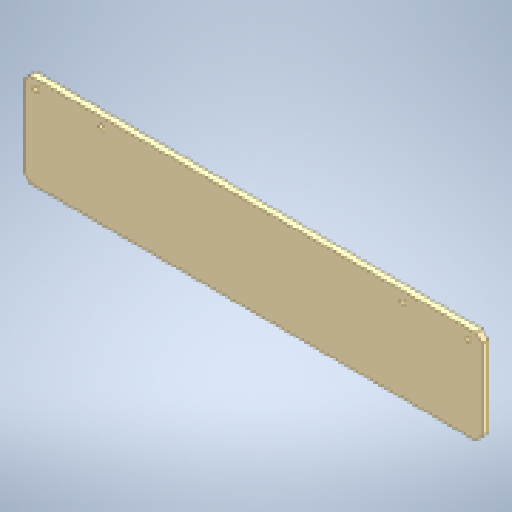
# Autodesk Inventor part: фанера_для_электр
Saved by Autodesk Inventor 2023.1 (Build 271208000, 208)
## iProperties
Created: 2026-01-13
Part Number: фанера_для_электр
Material: Типовые
Document SubType Name: Modeling
Designer: DELL
Density: 1 g/cm^3
Appearance: Бежевый
Author: DELL
Autodesk Inventor part; units mm, degrees
ref_plane "YZ Plane" through (0, 0, 0) normal (1, 0, 0) x (0, 1, 0)
ref_plane "XZ Plane" through (0, 0, 0) normal (0, 1, 0) x (-1, 0, 0)
ref_plane "XY Plane" through (0, 0, 0) normal (0, 0, 1) x (1, 0, 0)
sketch "Эскиз1" plane through (0, 0, 0) normal (0, 0, 1) x (1, 0, 0)
  line L0 (-286.7881, 32) -> (-6.2881, 32)
  line L1 (-6.2881, 32) -> (-6.2881, -25)
  line L2 (-6.2881, -25) -> (-286.7881, -25)
  line L3 (-286.7881, -25) -> (-286.7881, 32)
  line L4 (-286.7881, 32) -> (-6.2881, -25) construction
  line L5 (-6.2881, 32) -> (-286.7881, -25) construction
  point P0 (0, 0)
  point P1 (-146.5381, 3.5)
  dimension "d0" = 280.5
  dimension "d1" = 57
  constraints: 12 end point, 2 midpoint, 2 parallel, 1 horizontal, 1 perpendicular
  measures "d0" distance of L1.end L2.end
  measures "d1" distance of L0.end L1.end
extrude "Выдавливание1" add sketch "Эскиз1" along normal blind 4
sketch "Эскиз2" plane through (0, 0, 4) normal (0, 0, 1) x (1, 0, 0)
  circle A0 centre (-54.2881, 26.0225) radius 2.1 construction
  circle A1 centre (-14.2881, 26.0225) radius 2.1 construction
  circle A2 centre (-278.7881, 26.4) radius 2.1 construction
  circle A3 centre (-238.7881, 26.4) radius 2.1 construction
  circle A4 centre (-14.2881, 26.0225) radius 1.65
  circle A5 centre (-54.2881, 26.0225) radius 1.65
  circle A6 centre (-238.7881, 26.4) radius 1.65
  circle A7 centre (-278.7881, 26.4) radius 1.65
  point P0 (0, 0)
  dimension "d4" = 3.3
  dimension "d5" = 3.3
  dimension "d6" = 3.3
  dimension "d7" = 3.3
  constraints: 4 centre point, 4 coincident
  measures "d4" diameter of A4
  measures "d5" diameter of A5
  measures "d6" diameter of A6
  measures "d7" diameter of A7
extrude "Выдавливание2" cut sketch "Эскиз2" against normal blind 4
chamfer "Фаска1" distance 4 angle 45 4 edges at (-286.7881, 32, 2) (-286.7881, -25, 2) (-6.2881, -25, 2) (-6.2881, 32, 2)
